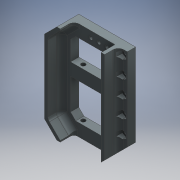
# Autodesk Inventor part: chassi_back_right
Saved by Autodesk Inventor 2016 (Build 200138000, 138)
## iProperties
Created: 2017-01-03
Part Number: chassi_back_right
Material: Generic
Document SubType Name: Modeling
Designer: hesaon
Density: 1 g/cm^3
Appearance: Default
Author: hesaon
Autodesk Inventor part; units mm, degrees
ref_plane "YZ Plane" through (0, 0, 0) normal (1, 0, 0) x (0, 1, 0)
ref_plane "XZ Plane" through (0, 0, 0) normal (0, 1, 0) x (-1, 0, 0)
ref_plane "XY Plane" through (0, 0, 0) normal (0, 0, 1) x (1, 0, 0)
sketch "Sketch1" plane through (0, 0, 0) normal (0, 1, 0) x (-1, 0, 0)
  line L0 (0, 117.0442) -> (0, 88.5)
  line L1 (0, 142.5) -> (-82.5, 142.5)
  line L2 (0, 0) -> (-60, 0)
  line L3 (-60, 0) -> (-82.5, 22.5)
  line L4 (-82.5, 142.5) -> (-82.5, 22.5)
  line L5 (-64.5, 124.5) -> (-7.4558, 124.5)
  line L6 (0, 88.5) -> (-64.5, 88.5)
  line L7 (-64.5, 29.9558) -> (-64.5, 70.5)
  line L8 (-64.5, 88.5) -> (-64.5, 124.5)
  line L9 (-52.5442, 18) -> (-64.5, 29.9558)
  line L10 (-45.5, 0) -> (0, 0)
  line L11 (-45.5, 0) -> (0, 0)
  line L12 (0, 0) -> (18, 18)
  line L13 (-7.4558, 18) -> (-52.5442, 18)
  line L14 (-64.5, 70.5) -> (0, 70.5)
  line L15 (0, 70.5) -> (0, 25.4558)
  line L16 (0, 25.4558) -> (-7.4558, 18)
  line L17 (0, 142.5) -> (18, 124.5)
  line L18 (18, 18) -> (18, 124.5)
  line L19 (0, 117.0442) -> (-7.4558, 124.5)
  point P0 (0, 0)
  dimension "d1" = 142.5
  dimension "d3" = 82.5
  dimension "d4" = 60
  dimension "d5" = 135
  dimension "d6" = 120
  dimension "d8" = 18
  dimension "d17" = 18
  dimension "d20" = 18
  dimension "d21" = 18
  dimension "d58" = 45.5
  dimension "d59" = 45.5
  dimension "d61" = 18
  dimension "d65" = 18
  dimension "d66" = 18
  dimension "d68" = 135
  dimension "d73" = 45
  dimension "d74" = 18
  dimension "d75" = 36
  dimension "d76" = 64.5
  dimension "d77" = 64.5
  dimension "d78" = 45
  dimension "d79" = 106.5
  constraints: 40 end point, 6 perpendicular, 4 horizontal, 4 vertical, 3 parallel, 1 coincident
  measures "d1" distance of L2.start L1.start
  measures "d3" distance of L1.start L1.end
  measures "d4" distance of L2.start L2.end
  measures "d5" angle of L2 L3
  measures "d6" distance of L3.end L1.end
  measures "d8" distance between parallel lines of L1 L5
  measures "d17" distance of L7.end L6.end
  measures "d20" distance between parallel lines of L4 L8
  measures "d21" distance between parallel lines of L3 L9
  measures "d58" distance of L2.start L10.start
  measures "d59" distance of L10.start L2.start
  measures "d61" distance between parallel lines of L2 L13
  measures "d65" distance between parallel lines of L16 L12
  measures "d66" distance between parallel lines of L4 L7
  measures "d68" angle of L13 L16
  measures "d73" angle of L0 L17
  measures "d74" distance between parallel lines of L17 L19
  measures "d75" distance between parallel lines of L5 L6
  measures "d76" distance between parallel lines of L8 L0
  measures "d77" distance between parallel lines of L7 L15
  measures "d78" angle of L12 L2
  measures "d79" distance of L17.end L12.end
extrude "Extrusion2" add sketch "Sketch1" along normal blind 12
sketch "Sketch7" plane through (0, 0, 0) normal (0, -1, 0) x (1, 0, 0)
  circle A0 centre (29.625, 133.5) radius 2.5
  circle A1 centre (41.25, 133.5) radius 2.5
  circle A2 centre (52.875, 133.5) radius 2.5
  line L0 (7.4558, 124.5) -> (64.5, 124.5) projected
  line L1 (0, 88.5) -> (0, 117.0442) projected
  line L2 (64.5, 124.5) -> (64.5, 88.5) projected
  point P0 (0, 0)
  dimension "d47" = 5
  dimension "d48" = 5
  dimension "d49" = 5
  dimension "d50" = 11.625
  dimension "d51" = 11.625
  dimension "d52" = 9
  dimension "d90" = 11.625
  constraints: 3 centre point, 2 horizontal alignment
  measures "d47" diameter of A0
  measures "d48" diameter of A1
  measures "d49" diameter of A2
  measures "d50" distance of A1.centre A0.centre
  measures "d51" distance of A1.centre A2.centre
  measures "d52" distance from line of L0 A0.centre
  measures "d90" distance from line of L2 A2.centre
extrude "Extrusion7" cut sketch "Sketch7" against normal up to next
sketch "Sketch8" plane through (60, 0, 0) normal (0, 0, -1) x (-1, 0, 0)
  line L0 (78, 0) -> (32.5, 0)
  line L1 (0, 0) -> (60, 0) projected
  circle A0 centre (47.5, 6) radius 3
  line L2 (32.5, 0) -> (32.5, 12)
  line L3 (0, 12) -> (60, 12) projected
  circle A1 centre (17.5, 6) radius 3
  dimension "d80" = 45.5
  dimension "d81" = 6
  dimension "d82" = 6
  dimension "d83" = 15
  dimension "d84" = 6
  dimension "d85" = 15
  dimension "d86" = 6
  constraints: 4 end point, 2 centre point, 2 point on line, 1 vertical
  measures "d80" distance of L0.start L0.end
  measures "d81" diameter of A0
  measures "d82" distance from line of L0 A0.centre
  measures "d83" distance from line of L2 A0.centre
  measures "d84" diameter of A1
  measures "d85" distance from line of A1.centre L2
  measures "d86" distance from line of L1 A1.centre
extrude "Extrusion8" cut sketch "Sketch8" against normal blind 88.5
sketch "Sketch9" plane through (0, 0, 0) normal (0, -1, 0) x (1, 0, 0)
  circle A0 centre (75.5, 35) radius 3
  line L0 (82.5, 142.5) -> (82.5, 22.5) projected
  circle A1 centre (75.5, 60) radius 3
  circle A2 centre (75.5, 85) radius 3
  circle A3 centre (75.5, 110) radius 3
  circle A4 centre (75.5, 135) radius 3
  point P0 (0, 0)
  dimension "d91" = 6
  dimension "d92" = 7
  dimension "d93" = 12.5
  dimension "d94" = 6
  dimension "d95" = 25
  dimension "d96" = 6
  dimension "d97" = 25
  dimension "d98" = 6
  dimension "d99" = 25
  dimension "d100" = 6
  dimension "d101" = 25
  constraints: 5 centre point, 4 vertical alignment
  measures "d91" diameter of A0
  measures "d92" distance from line of L0 A0.centre
  measures "d93" vertical distance of A0.centre L0.end
  measures "d94" diameter of A1
  measures "d95" distance of A1.centre A0.centre
  measures "d96" diameter of A2
  measures "d97" distance of A2.centre A1.centre
  measures "d98" diameter of A3
  measures "d99" distance of A2.centre A3.centre
  measures "d100" diameter of A4
  measures "d101" distance of A4.centre A3.centre
extrude "Extrusion9" cut sketch "Sketch9" against normal up to next
sketch "Sketch11" plane through (0, 0, 0) normal (0, -1, 0) x (1, 0, 0)
  circle A0 centre (75.5, 135) radius 3 projected
  line L0 (80.7, 131.9978) -> (75.5, 128.9956)
  line L1 (75.5, 128.9956) -> (70.3, 131.9978)
  line L2 (70.3, 131.9978) -> (70.3, 138.0022)
  line L3 (70.3, 138.0022) -> (75.5, 141.0044)
  line L4 (75.5, 141.0044) -> (80.7, 138.0022)
  line L5 (80.7, 138.0022) -> (80.7, 131.9978)
  line L6 (82.5, 142.5) -> (82.5, 22.5) projected
  circle A1 centre (75.5, 110) radius 3 projected
  line L7 (75.5, 116.0044) -> (80.6999, 113.0022)
  line L8 (80.6999, 113.0022) -> (80.6999, 106.9978)
  line L9 (80.6999, 106.9978) -> (75.5, 103.9956)
  line L10 (75.5, 103.9956) -> (70.3001, 106.9978)
  line L11 (70.3001, 106.9978) -> (70.3001, 113.0022)
  line L12 (70.3001, 113.0022) -> (75.5, 116.0044)
  circle A2 centre (75.5, 85) radius 3 projected
  line L13 (75.5, 91.0044) -> (80.7, 88.0022)
  line L14 (80.7, 88.0022) -> (80.7, 81.9978)
  line L15 (80.7, 81.9978) -> (75.5, 78.9956)
  line L16 (75.5, 78.9956) -> (70.3, 81.9978)
  line L17 (70.3, 81.9978) -> (70.3, 88.0022)
  line L18 (70.3, 88.0022) -> (75.5, 91.0044)
  circle A3 centre (75.5, 60) radius 3 projected
  line L19 (80.7, 63.0022) -> (80.7, 56.9978)
  line L20 (80.7, 56.9978) -> (75.5, 53.9956)
  line L21 (75.5, 53.9956) -> (70.3, 56.9978)
  line L22 (70.3, 56.9978) -> (70.3, 63.0022)
  line L23 (70.3, 63.0022) -> (75.5, 66.0044)
  line L24 (75.5, 66.0044) -> (80.7, 63.0022)
  circle A4 centre (75.5, 35) radius 3 projected
  line L25 (75.5, 41.0044) -> (80.7, 38.0022)
  line L26 (80.7, 38.0022) -> (80.7, 31.9978)
  line L27 (80.7, 31.9978) -> (75.5, 28.9956)
  line L28 (75.5, 28.9956) -> (70.3, 31.9978)
  line L29 (70.3, 31.9978) -> (70.3, 38.0022)
  line L30 (70.3, 38.0022) -> (75.5, 41.0044)
  point P0 (0, 0)
  dimension "d112" = 10.4
  dimension "d113" = 10.3999
  dimension "d114" = 10.4
  dimension "d118" = 10.4
  dimension "d119" = 10.4
  constraints: 60 end point, 5 coincident, 5 parallel, 65 other
  measures "d112" distance between parallel lines of L2 L5
  measures "d113" distance between parallel lines of L11 L8
  measures "d114" distance between parallel lines of L14 L17
  measures "d118" distance between parallel lines of L22 L19
  measures "d119" distance between parallel lines of L29 L26
extrude "Extrusion11" cut sketch "Sketch11" against normal blind 5
sketch "Sketch12" plane through (0, 0, 0) normal (0, -1, 0) x (1, 0, 0)
  line L0 (0, 142.5) -> (82.5, 142.5) projected
  line L1 (82.5, 22.5) -> (60, 0) projected
  line L2 (64.5, 142.5) -> (69.5, 142.5)
  line L3 (69.5, 142.5) -> (69.5, 9.5)
  line L4 (64.5, 9.5) -> (64.5, 142.5)
  line L5 (64.5, 9.5) -> (64.5, 4.5)
  point P0 (0, 0)
  dimension "d122" = 5
  dimension "d123" = 5
  dimension "d124" = 4.5
  constraints: 8 end point, 3 point on line, 1 horizontal, 1 parallel, 1 perpendicular, 1 vertical
  measures "d122" distance of L3.end L4.start
  measures "d123" distance between parallel lines of L3 L4
  measures "d124" vertical distance of L5.end point (0, 0)
extrude "Extrusion12" add sketch "Sketch12" along normal blind 20
fillet "Fillet1" radius 8 1 edges at (69.5, 0, 76)
sketch "Sketch13" plane through (0, 0, 0) normal (0, -1, 0) x (1, 0, 0)
  line L0 (60, 0) -> (0, 0) projected
  line L1 (0, 0) -> (5, 0)
  line L2 (5, 0) -> (5, 2.0711)
  line L3 (5, 2.0711) -> (-13, 20.0711)
  line L4 (-18, 18) -> (-18, 124.5) projected
  line L5 (0, 0) -> (-18, 18)
  line L6 (-18, 18) -> (-18, 124.5)
  line L7 (-18, 124.5) -> (0, 142.5) projected
  line L8 (0, 142.5) -> (5, 142.5)
  line L9 (0, 142.5) -> (64.5, 142.5) projected
  line L10 (5, 140.4289) -> (-13, 122.4289)
  line L11 (5, 140.4289) -> (5, 142.5)
  line L12 (-13, 20.0711) -> (-13, 122.4289)
  line L13 (-18, 124.5) -> (0, 142.5)
  line L14 (5, 140.4289) -> (5, 142.5)
  line L15 (0, 0) -> (-18, 18) projected
  dimension "d131" = 5
  dimension "d132" = 5
  dimension "d133" = 5
  dimension "d134" = 5
  dimension "d135" = 5
  constraints: 22 end point, 3 parallel, 3 perpendicular, 2 point on line, 1 collinear, 1 vertical
  measures "d131" distance between parallel lines of L12 L4
  measures "d132" distance between parallel lines of L7 L10
  measures "d133" distance of L8.end L7.end
  measures "d134" distance between parallel lines of L3 L5
  measures "d135" distance of L1.end L0.end
extrude "Extrusion13" add sketch "Sketch13" along normal blind 20
fillet "Fillet2" radius 8 1 edges at (-13, 0, 71.25)
fillet "Fillet3" radius 8 1 edges at (0, 0, 7.0711)
fillet "Fillet4" radius 8 1 edges at (0, 0, 135.4289)
fillet "Fillet5" radius 5.25 1 edges at (5, 0, 6.6924)
fillet "Fillet6" radius 8 1 edges at (5, 0, 135.8076)
body "Solid2"
